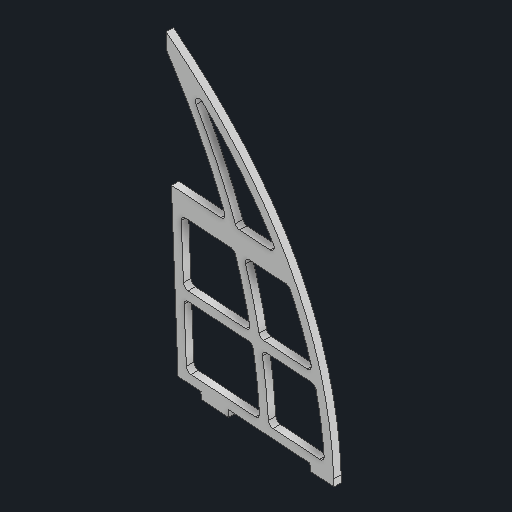
# Autodesk Inventor part: sponson_spanner_side
Saved by Autodesk Inventor 2023 (Build 270158030, 158C)
## iProperties
Created: 2022-03-22
Part Number: sponson_spanner_side
Material: Generic
Document SubType Name: Modeling
Designer: kardo
Density: 1 g/cm^3
Appearance: Default
Mass: 7.03333 g
Surface Area: 74.9143 cm^2
Volume: 7.03333 cm^3
Author: kardo
Autodesk Inventor part; units mm, degrees
ref_plane "YZ Plane" through (0, 0, 0) normal (1, 0, 0) x (0, 1, 0)
ref_plane "XZ Plane" through (0, 0, 0) normal (0, 1, 0) x (-1, 0, 0)
ref_plane "XY Plane" through (0, 0, 0) normal (0, 0, 1) x (1, 0, 0)
derived "surface_body.ipt"
sketch "sk_rail_sponson_side" plane through (81.12, 255, 36.448) normal (0.06099, 0.0391867, -0.9973689) x (0.2816917, -0.9592867, -0.0204648)
  line L0 (265.8225, 0) -> (150.2798, -33.9898)
  spline S0 degree 2 poles (150.2798, -33.9898) (71.6973, -57.1068) (0, 0) knots 0 0 0 1 1 1
  point P0 (222.5132, 151.5365)
ref_plane "plane_tunnel_right" through (81.12, 0, 0) normal (1, 0, 0) x (0, 1, 0)
ref_plane "plane_sponson_side" through (81.12, 255, 36.448) normal (0.06099, 0.0391867, -0.9973689) x (0.2816917, -0.9592867, -0.0204648)
sketch "sk_rail_sponson_tunnel" plane through (81.12, 0, 0) normal (1, 0, 0) x (0, 1, 0)
  line L0 (0, 0) -> (122.4, 9.6331)
  line L1 (111.1171, 152.996) -> (142.2856, -243.0375) construction
  spline S0 degree 2 poles (122.4, 9.6331) (190.08, 14.9596) (255, 36.448) knots 0 0 0 1 1 1
sketch "sk_rail_sponson_bottom" plane through (126.048, 0, 0) normal (0.341579, -0.07374, 0.9369558) x (-0.1718217, 0.9752166, 0.139391)
  line L0 (120.7093, -22.4461) -> (0, 0)
  line L1 (389.6045, -72.4475) -> (-475.366, 88.395) construction
  line L2 (163.4334, 207.3137) -> (92.7222, -172.9535) construction
  spline S0 degree 2 poles (120.7093, -22.4461) (192.8116, -35.8536) (261.4804, 0) knots 0 0 0 1 1 1
  point P0 (21.6578, 116.4701)
sketch "sk_rail_top_tunnel" plane through (81.12, 0, 0) normal (1, 0, 0) x (0, 1, 0)
  line L0 (255, 107.6209) -> (255, -224.5198) construction
  line L1 (0, 107.6209) -> (0, -224.5198) construction
  line L2 (-345, 107.6209) -> (-345, -224.5198) construction
  line L3 (-345, 0) -> (0, 0) construction
  line L4 (-172.5, 48.8998) -> (-172.5, 0) construction
  line L5 (0, 52.89) -> (37.026, 52.89) construction
  line L6 (37.026, 52.89) -> (80.784, 47.0555) construction
  line L7 (80.784, 47.0555) -> (112.2, 37.536) construction
  line L8 (112.2, 107.6209) -> (112.2, -224.5198) construction
  line L9 (0, 52.89) -> (255, 52.89) construction
  line L10 (-469.9275, 0) -> (379.2584, 0) construction
  spline S0 degree 3 poles (0, 52.89) (92.8353, 52.89) (195.0311, 49.5089) (255, 36.448) knots 0 0 0 0 1 1 1 1
  spline S1 degree 3 poles (0, 52.89) (37.026, 52.89) (80.784, 47.0555) (112.2, 37.536) knots 1 1 1 1 2 2 2 2
  spline S2 degree 4 poles (-345, 37.3935) (-258.8686, 45.1235) (-172.5923, 49.7074) (-86.3167, 52.89) (0, 52.89) knots 0 0 0 0 0 1 1 1 1 1
  point P0 (153, 48.7795)
  point P1 (112.2, 28.832)
  point P2 (-230.0001, 45.8224)
  point P3 (-114.9999, 50.9907)
sketch "sk_section_sponson_break" plane through (0, 122.4, 9.6331) normal (0, 0.9969173, 0.0784591) x (-1, 0, 0)
  line L0 (-268.0445, -51.607) -> (63.6955, 68.9601) construction
  line L1 (-81.12, -266.2886) -> (-81.12, 157.0776) construction
  arc A0 (-81.12, 41.081) -> (-156, 26.184) centre (-72.7535, -196.6143) ccw construction
  arc A1 (-54.6, 54.2323) -> (-156, 30.9124) centre (-53.2835, -183.6066) ccw construction
  spline S0 degree 2 poles (-54.6, 54.2323) (-107.2974, 54.2323) (-156, 30.9124) knots 0 0 0 1 1 1
  spline S1 degree 2 poles (-156, 26.184) (-120.0091, 39.6317) (-81.12, 41.081) knots 0 0 0 1 1 1
  point P0 (0, 0)
ref_plane "plane_sponson_break" through (0, 122.4, 9.6331) normal (0, 0.9969173, 0.0784591) x (-1, 0, 0)
derived "parameters_frame.ipt"
derived "stencil_frame.ipt"
sketch "sk_joint_locations" plane through (81.12, 0, 0) normal (1, 0, 0) x (0, 1, 0)
  line L0 (0, 0) -> (122.4, 9.6331) construction
  line L1 (36.465, 28.832) -> (112.2, 28.832) construction
  arc A0 (36.465, 28.832) -> (11.22, 28.376) centre (36.465, -670.197) ccw construction
  line L2 (-241.5001, 19.2432) -> (11.22, 28.376) construction
  line L3 (-345, 16.32) -> (-262.2001, 18.586) construction
  arc A1 (-262.2001, 18.586) -> (-241.5001, 19.2432) centre (-326.8578, 2381.2399) ccw construction
  line L4 (-122.4795, 3121.122) -> (270.8781, -1876.9598) construction
  line L5 (-230.0001, 3089.1136) -> (-230.0001, -1866.0023) construction
  line L6 (-114.9999, 3089.1136) -> (-114.9999, -1866.0023) construction
  line L7 (-345, 3089.1136) -> (-345, -1866.0023) construction
  line L8 (0, 3089.1136) -> (0, -1866.0023) construction
  line L9 (529.622, 47.2379) -> (-602.608, 2.7525) construction
  line L10 (-673.1615, -36.5999) -> (647.9226, 67.3717) construction
  line L11 (189.4528, 29.5173) -> (189.1111, 38.2146) construction
  line L12 (201.105, 36.5853) -> (201.7901, 27.8813) construction
  line L13 (0, 14.144) -> (121.9006, 15.9783) construction
  line L14 (-230.0001, 45.8224) -> (-230.0001, 19.6588) construction
  line L15 (-345, 37.3935) -> (-345, 16.32) construction
  line L16 (-114.9999, 50.9907) -> (-114.9999, 23.8147) construction
  line L17 (0, 52.89) -> (0, 27.9705) construction
  line L18 (119.1768, 50.5875) -> (119.7216, 43.6656) construction
  line L19 (120.2663, 36.7438) -> (119.7216, 43.6656) construction
  line L20 (120.2663, 36.7438) -> (120.8111, 29.822) construction
  line L21 (120.8111, 29.822) -> (121.3559, 22.9001) construction
  line L22 (121.3559, 22.9001) -> (121.9006, 15.9783) construction
  line L23 (0, 14.144) -> (0, 0) construction
  line L24 (112.2, 37.536) -> (112.2, 28.832) construction
  line L25 (112.2, 35.848) -> (112.2, 30.52) construction
  spline S0 degree 4 poles (-345, 37.3935) (-258.8686, 45.1235) (-172.5923, 49.7074) (-86.3167, 52.89) (0, 52.89) knots 0 0 0 0 0 1 1 1 1 1
  spline S1 degree 3 poles (0, 52.89) (92.8353, 52.89) (195.0311, 49.5089) (255, 36.448) knots 0 0 0 0 1 1 1 1
  spline S2 degree 2 poles (122.4, 9.6331) (190.08, 14.9596) (255, 36.448) knots 0 0 0 1 1 1
  point P0 (-122.4795, 3121.122)
  point P1 (270.8781, -1876.9598)
  point P2 (189.282, 33.8659)
  point P3 (201.4475, 32.2333)
  point P4 (134.9575, 11.3411)
  point P5 (-345, 26.8568)
  point P6 (-230.0001, 32.7406)
  point P7 (-114.9999, 37.4027)
  point P8 (0, 40.4303)
  point P9 (112.2, 33.184)
sketch "sk_spanner_joints_locations" plane through (0, 122.4, 9.6331) normal (0, 0.9969173, 0.0784591) x (-1, 0, 0)
  line L0 (328.7115, -3.4565) -> (-466.2934, 45.1587) construction
  line L1 (-867.9776, -269.6459) -> (1175.5999, 473.0692) construction
  line L2 (-94.4551, 22.4205) -> (-92.9508, 12.0288) construction
  line L3 (-94.4551, 22.4205) -> (-68.6928, 20.8451) construction
  line L4 (-92.9508, 12.0288) -> (-68.6928, 20.8451) construction
  point P0 (0, 0)
  point P1 (-126.048, 0)
  point P2 (-156, 26.184)
  point P3 (-143.691, 25.4313)
  point P4 (-106.7641, 23.1732)
  point P5 (-101.2251, 9.0216)
  point P6 (-117.7737, 3.0072)
ref_plane "plane_stringer_outer" through (84.12, 0, 0) normal (1, 0, 0) x (0, 1, 0)
sketch "sk_corner_offset" plane through (0, 122.4, 9.6331) normal (0, 0.9969173, 0.0784591) x (-1, 0, 0)
  spline S0 degree 2 poles (-156, 26.184) (-120.0091, 39.6317) (-81.12, 41.081) knots 0 0 0 1 1 1 construction
  line L0 (-156, 26.184) -> (-126.048, 0) construction
  line L1 (-154.4608, 25.9011) -> (-125.5215, 0.6023) construction
  line L2 (-125.5215, 0.6023) -> (-126.048, 0) construction
  spline S1 degree 5 poles (-154.4608, 25.9011) (-140.3656, 31.0778) (-125.865, 35.1515) (-111.0589, 38.0354) (-96.0956, 39.7222) (-81.0902, 40.2816) knots 0 0 0 0 0 0 1 1 1 1 1 1 construction
  point P0 (0, 0)
  dimension "d9" = 0.8
  dimension "d10" = 0.8
  constraints: 6 end point, 1 coincident, 1 parallel, 1 perpendicular, 3 other
  measures "d10" distance between parallel lines of L1 L0
sketch "sk_tip_offset" plane through (81.12, 0, 0) normal (1, 0, 0) x (0, 1, 0)
  spline S0 degree 3 poles (0, 52.89) (92.8353, 52.89) (195.0311, 49.5089) (255, 36.448) knots 0 0 0 0 1 1 1 1 construction
  spline S1 degree 2 poles (122.4, 9.6331) (190.08, 14.9596) (255, 36.448) knots 0 0 0 1 1 1 construction
  spline S2 degree 5 poles (0, 52.09) (14.1126, 52.09) (28.2252, 52.0249) (42.3374, 51.8877) (70.3021, 51.4557) (98.2587, 50.655) (112.105, 50.1551) (138.5853, 48.9703) (165.0353, 47.2425) (177.6496, 46.2711) (200.1482, 44.2213) (222.5619, 41.3963) (232.3977, 39.9657) (242.2024, 38.3071) (251.9318, 36.2831) knots 0 0 0 0 0 0 0.279151 0.279151 0.279151 0.553204 0.553204 0.553204 0.803431 0.803431 0.803431 1 1 1 1 1 1 construction
  spline S3 degree 4 poles (122.3372, 10.4306) (155.3484, 13.0285) (188.1618, 18.2132) (220.4424, 26.04) (251.9318, 36.2832) knots 0 0 0 0 0 1 1 1 1 1 construction
  point P0 (0, 0)
  dimension "d7" = 0.8
  dimension "d8" = 0.8
  constraints: 1 coincident, 6 other
sketch "sk_sponson_spanner_side_base" plane through (81.12, 255, 36.448) normal (0.06099, 0.0391867, -0.9973689) x (0.2816917, -0.9592867, -0.0204648)
  spline S0 degree 2 poles (150.2798, -33.9898) (71.6973, -57.1068) (0, 0) knots 0 0 0 1 1 1 construction
  line L0 (132.7366, 25.1218) -> (129.7906, 35.0482)
  line L1 (136.2452, 13.2995) -> (146.7712, -22.1675)
  line L2 (146.7712, -22.1675) -> (149.6472, -21.3139)
  line L3 (149.6472, -21.3139) -> (152.7158, -31.6538)
  line L4 (136.2452, 13.2995) -> (139.1213, 14.153)
  line L5 (139.1213, 14.153) -> (135.6126, 25.9753)
  line L6 (135.6126, 25.9753) -> (132.7366, 25.1218)
  line L7 (748.8189, 217.151) -> (-250.2454, -76.7489) projected
  line L8 (152.7158, -31.6538) -> (149.8307, -32.5025)
  line L9 (265.8225, 0) -> (150.2798, -33.9898) construction
  spline S1 degree 2 poles (2.9467, 0.8697) (72.9898, -55.1072) (149.8307, -32.5025) knots 0 0 0 1 1 1
  point P0 (222.5132, 151.5365)
  point P1 (63.0953, 18.5611)
  point P2 (99.6986, 28.3676)
  point P3 (2.9047, -2.2785)
  point P4 (5.8476, -1.4127)
  dimension "d3" = 3
  constraints: 16 end point, 4 parallel, 2 collinear, 2 perpendicular, 1 point on line, 3 other
  measures "d3" distance between parallel lines of L5 L1
extrude "thicken" add sketch "sk_sponson_spanner_side_base" along normal blind 3
sketch "sk_cut_weight" plane through (81.12, 255, 36.448) normal (0.06099, 0.0391867, -0.9973689) x (0.2816917, -0.9592867, -0.0204648)
  line L0 (132.7366, 25.1218) -> (129.7906, 35.0482) construction
  line L1 (136.2452, 13.2995) -> (146.7712, -22.1675) construction
  spline S0 degree 2 poles (2.9467, 0.8697) (72.9898, -55.1072) (149.8307, -32.5025) knots 0 0 0 1 1 1 construction
  line L2 (63.0953, 18.5611) -> (77.9952, -32.0887) construction
  line L3 (70.8285, 13.5335) -> (77.6368, -9.6102)
  line L4 (61.0655, 14.831) -> (68.1742, -9.3339)
  line L5 (61.0655, 14.831) -> (12.7084, 0.6055)
  line L6 (70.8285, 13.5335) -> (127.0913, 30.0847)
  line L7 (127.0913, 30.0847) -> (136.5255, -1.7037)
  line L8 (78.8149, -13.6151) -> (84.6068, -33.3034)
  line L9 (69.3692, -13.3961) -> (74.6501, -31.3477)
  line L10 (137.6637, -5.539) -> (144.8488, -29.7492)
  line L11 (98.9599, 21.8091) -> (115.5802, -34.6888) construction
  line L12 (105.6271, -7.9416) -> (97.0412, 21.2447)
  line L13 (100.8786, 22.3735) -> (109.6358, -7.395)
  line L14 (110.7757, -11.2702) -> (117.6203, -34.5371)
  line L15 (106.7703, -11.8278) -> (113.5315, -34.8114)
  line L16 (748.8189, 217.151) -> (-250.2454, -76.7489) construction
  spline S1 degree 2 poles (141.5082, -4.434) (74.9073, -24.1999) (5.8476, -1.4127) knots 0 0 0 1 1 1
  spline S2 degree 5 poles (17.3723, -4.9239) (23.8633, -9.4451) (30.5645, -13.6647) (37.4799, -17.5368) (53.4513, -25.3109) (70.365, -30.7939) (79.9803, -33.0268) (98.8488, -35.6296) (117.874, -34.965) (127.0046, -33.8874) (136.0083, -32.123) (144.8488, -29.7492) knots 0 0 0 0 0 0 0.294267 0.294267 0.294267 0.659481 0.659481 0.659481 1 1 1 1 1 1
  spline S3 degree 5 poles (136.5254, -1.7037) (124.4108, -5.0682) (112.0625, -7.5902) (99.5423, -9.1939) (74.3937, -10.4895) (49.3272, -8.0803) (36.9222, -5.9766) (24.7034, -3.0528) (12.7084, 0.6055) knots 0 0 0 0 0 0 0.500649 0.500649 0.500649 1 1 1 1 1 1
  point P0 (222.5132, 151.5365)
  dimension "d11" = 4
  dimension "d20" = 4
  dimension "d14" = 3
  dimension "d15" = 6
  dimension "d16" = 4
  dimension "d19" = 4
  dimension "d21" = 4
  constraints: 28 end point, 6 collinear, 5 parallel, 3 point on line, 2 midpoint, 2 perpendicular, 28 other
  measures "d14" distance between parallel lines of L2 L4
  measures "d15" distance between parallel lines of L2 L3
  measures "d16" distance between parallel lines of L1 L7
  measures "d19" distance between parallel lines of L13 L12
  measures "d21" distance between parallel lines of L16 L6
extrude "cut_weight" cut sketch "sk_cut_weight" along normal through all both and the other way through all contours L6 L12 S3 L3 | L6 L7 S3 L13 | L4 S3 L5 | S1 L15 S2 L8 | L9 S2 S1 | S1 L10 S2 L14
fillet "rounding" radius 2 21 edges at (88.204, 124.727, 30.2588) (125.2941, 124.5491, 32.5199) (122.6137, 155.9437, 33.5895) (88.204, 156.0263, 31.4885) (113.5798, 192.2608, 34.464) (88.204, 152.0294, 31.3315) (88.204, 183.3286, 32.5613) (116.4503, 183.2608, 34.2859) (90.8201, 239.771, 34.9389) (123.208, 151.9454, 33.4687) (112.2835, 183.2708, 34.0315) (136.9347, 183.2117, 35.5366) (119.1762, 151.9551, 33.2226) (147.4157, 151.8873, 34.9468) (132.2573, 192.216, 35.6043) (150.501, 124.4282, 34.0566) (146.5265, 155.8864, 35.0495) (121.3009, 124.5683, 32.2765) (109.3534, 192.2709, 34.2059) (84.2115, 242.6984, 34.6498) (118.5704, 155.9534, 33.3426)
equation "\"d9\" = shell_thickness"
equation "\"d10\" = shell_thickness"
equation "\"d7\" = shell_thickness"
equation "\"d8\" = shell_thickness"
equation "\"d3\" = bulkhead_thickness"
equation "\"d5\" = bulkhead_thickness"
equation "\"d11\" = bulkhead_inset"
equation "\"d20\" = bulkhead_inset"
equation "\"d14\" = bulkhead_thickness"
equation "\"d15\" = 2 * bulkhead_thickness"
equation "\"d16\" = bulkhead_inset"
equation "\"d19\" = bulkhead_inset"
equation "\"d21\" = bulkhead_inset"
equation "\"d25\" = 0.5 * bulkhead_inset"
equation "\"d4\" = stringer_thickness"
equation "\"shell_thickness\" = 0.8"
equation "\"bulkhead_thickness\" = 3"
equation "\"bulkhead_inset\" = 4"
equation "\"stringer_thickness\" = 3"
body "Solid1"
